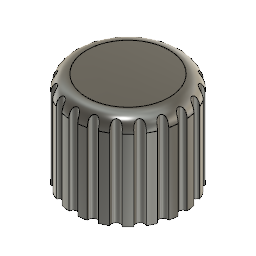
Macap digital knob (Autodesk Fusion 360 design; units mm, degrees)
Autodesk Fusion 360 part; units mm, degrees
sketch "Sketch1" plane through (0, 0, 0) normal (0, 0, 1) x (1, 0, 0)
  circle A0 centre (0, 0) radius 7
  dimension "d1" = 14
  constraint coincident A0.centre origin
  measures "d1" diameter of A0
extrude "Extrude1" add sketch "Sketch1" along normal blind 12
fillet "Fillet1" radius 1.75 1 edges at (-6.5263, -2.5313, 12)
sketch "Sketch2" plane through (0, 0, 0) normal (0, 0, -1) x (1, 0, 0)
  circle A0 centre (0, 0) radius 7
  circle A1 centre (0, 0) radius 7
  circle A2 centre (0, 0) radius 6
  circle A3 centre (0, 0) radius 7
  line L0 (0, 0) -> (0, 0.2) construction
  line L1 (0, 0.2) -> (0, 7) construction
  line L2 (0, 6) -> (0.65, 6) construction
  line L3 (0, 7) -> (0.6591, 6.9689) construction
  line L4 (0.65, 6) -> (0.65, 6.9845) construction
  line L5 (0.65, 6.4922) -> (0, 6.4922) construction
  circle A4 centre (0, 7) radius 0.5657
  circle A5 centre (-2.1631, 6.6574) radius 0.5657
  circle A6 centre (-4.1145, 5.6631) radius 0.5657
  circle A7 centre (-5.6631, 4.1145) radius 0.5657
  circle A8 centre (-6.6574, 2.1631) radius 0.5657
  circle A9 centre (-7, 0) radius 0.5657
  circle A10 centre (-6.6574, -2.1631) radius 0.5657
  circle A11 centre (-5.6631, -4.1145) radius 0.5657
  circle A12 centre (-4.1145, -5.6631) radius 0.5657
  circle A13 centre (-2.1631, -6.6574) radius 0.5657
  circle A14 centre (0, -7) radius 0.5657
  circle A15 centre (2.1631, -6.6574) radius 0.5657
  circle A16 centre (4.1145, -5.6631) radius 0.5657
  circle A17 centre (5.6631, -4.1145) radius 0.5657
  circle A18 centre (6.6574, -2.1631) radius 0.5657
  circle A19 centre (7, 0) radius 0.5657
  circle A20 centre (6.6574, 2.1631) radius 0.5657
  circle A21 centre (5.6631, 4.1145) radius 0.5657
  circle A22 centre (4.1145, 5.6631) radius 0.5657
  circle A23 centre (2.1631, 6.6574) radius 0.5657
  dimension "d6" = 1
  dimension "d8" = 360
  constraint concentric A1 A2
  constraint concentric A2 A3
  constraint coincident A0.centre A1.centre
  constraint vertical L0
  constraint coincident A1 L1.end
  constraint parallel L0 L1
  constraint coincident L1 L2.start
  constraint coincident A2 L2.start
  constraint perpendicular L1 L2
  constraint coincident A3 L3.end
  constraint perpendicular L2 L4
  constraint midpoint L4 L5.start
  constraint coincident L1 L5.end
  constraint perpendicular L1 L5
  constraint coincident L1.end L3.start
  measures "d6" distance of A0 A2
extrude "Extrude2" cut sketch "Sketch2" against normal up to surface (12 mm away) contours A0 A1 A3 A19 | A0 A1 A3 A20 | A0 A1 A3 A18 | A0 A1 A3 A21 | A0 A1 A3 A17 | A0 A1 A3 A22 | A0 A1 A3 A16 | A0 A1 A3 A23 | A0 A1 A3 A15 | A0 A1 A3 A4 | A0 A1 A3 A14 | A0 A1 A3 A5 | A0 A1 A3 A13 | A0 A1 A3 A6 | A0 A1 A3 A12 | A0 A1 A3 A7 | A0 A1 A3 A11 | A0 A1 A3 A8 | A0 A1 A3 A10 | A0 A1 A3 A9 picked at (6.823, -0.1301) picked at (6.4727, 2.1175) picked at (6.4727, -2.1175) picked at (5.5015, 4.0141) picked at (5.5015, -4.0141) picked at (4.0141, 5.5015) picked at (4.0141, -5.5015) picked at (2.0914, 6.4812) picked at (2.0914, -6.4812) picked at (-0.0137, 6.8102) picked at (-0.0137, -6.8102) picked at (-2.1158, 6.4731) picked at (-2.1158, -6.4731) picked at (-3.9923, 5.5173) picked at (-3.9923, -5.5173) picked at (-5.5036, 4.0109) picked at (-5.5036, -4.0109) picked at (-6.4748, 2.1098) picked at (-6.4748, -2.1098) picked at (-6.8097, 0)
sketch "Sketch3" plane through (0, 0, 0) normal (0, 0, 1) x (1, 0, 0)
  circle A0 centre (0, 0) radius 6
  dimension "d11" = 12
  constraint coincident A0.centre origin
  measures "d11" diameter of A0
extrude "Extrude3" cut sketch "Sketch3" along normal blind 2.4
sketch "Sketch4" plane through (0, 0, 2.4) normal (0, 0, -1) x (1, 0, 0)
  circle A0 centre (0, 0) radius 6
  circle A1 centre (0, 0) radius 3.5
  dimension "d14" = 7
  constraint concentric A0 A1
  measures "d14" diameter of A1
extrude "Extrude4" cut sketch "Sketch4" against normal blind 1.8 contours A1
sketch "Sketch5" plane through (0, 0, 4.2) normal (0, 0, -1) x (1, 0, 0)
  circle A0 centre (0, 0) radius 3.5
  circle A1 centre (0, 0) radius 3.5
  circle A2 centre (0, 0) radius 3.15
  line L0 (1.65, 4.5) -> (1.65, -4.3)
  line L1 (3.15, 4.1) -> (3.15, -3.8) construction
  dimension "d17" = 6.3
  dimension "d18" = 1.5
  constraint concentric A1 A2
  constraint vertical L0
  constraint vertical L1
  constraint tangent A2 L1
  measures "d17" diameter of A2
  measures "d18" distance of L0 L1
extrude "Extrude5" cut sketch "Sketch5" against normal up to surface (5.8 mm away) contours A2 L0 picked at (0.0528, -0.0768)
named bodies: "Macap digital knob"
